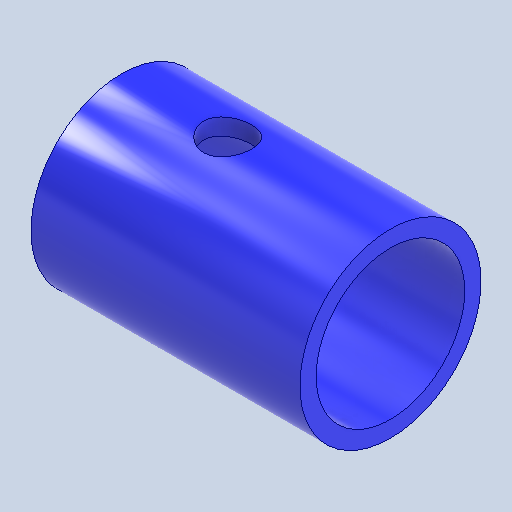
# Autodesk Inventor part: roller-hand-v1-3DP-shaft-spesa
Saved by Autodesk Inventor 2025.1 (Build 291241000, 241)
## iProperties
Created: 2024-10-01
Part Number: roller-hand-v1-3DP-shaft-spesa
Material: ABS プラスチック
Document SubType Name: Modeling
Designer: haruy
Density: 1.06 g/cm^3
Appearance: 青 - 壁塗料 - 光沢
Author: haruy
Autodesk Inventor part; units mm, degrees
ref_plane "YZ Plane" through (0, 0, 0) normal (1, 0, 0) x (0, 1, 0)
ref_plane "XY Plane" through (0, 0, 0) normal (0, 0, 1) x (1, 0, 0)
sketch "スケッチ1" plane through (0, 0, 0) normal (1, 0, 0) x (0, 1, 0)
  circle A0 centre (0, 0) radius 5.25
  circle A1 centre (0, 0) radius 6.4
  dimension "d0" = 10.5
  dimension "d1" = 12.8
  constraints: 2 centre point, 2 coincident
  measures "d0" diameter of A0
  measures "d1" diameter of A1
extrude "押し出し1" add sketch "スケッチ1" along normal blind 19
ref_plane "作業平面1" through (0, 6.4, 0) normal (0, 1, 0) x (-1, 0, 0)
sketch "スケッチ2" plane through (0, 6.4, 0) normal (0, 1, 0) x (-1, 0, 0)
  line L0 (0, 6.4) -> (0, -6.4) projected
  point P0 (0, 0)
  point P1 (-7.5, 0)
  dimension "d4" = 7.5
  measures "d4" distance from line of point (-7.5, 0) L0
hole "穴1" at (7.5, 6.4, 0) direction (0, -1, 0) diameter 3.4 end through all
